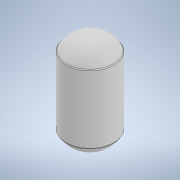
# Autodesk Inventor part: 80. Плунжер стопорный штоков (размер)
Saved by Autodesk Inventor 2021 (Build 250183000, 183)
## iProperties
Created: 2021-03-15
Part Number: 80. Плунжер стопорный штоков (размер)
Material: Типовые
Document SubType Name: Modeling
Designer: Данил
Density: 1 g/cm^3
Appearance: По умолчанию
Author: Данил
Autodesk Inventor part; units mm, degrees
ref_plane "YZ Plane" through (0, 0, 0) normal (1, 0, 0) x (0, 1, 0)
ref_plane "XZ Plane" through (0, 0, 0) normal (0, 1, 0) x (-1, 0, 0)
ref_plane "XY Plane" through (0, 0, 0) normal (0, 0, 1) x (1, 0, 0)
sketch "Эскиз1" plane through (0, 0, 0) normal (0, 0, 1) x (1, 0, 0)
  line L0 (0, 8) -> (0, -8)
  arc A0 (0, -8) -> (3.8971, -5.75) centre (0, -3.5) ccw
  line L1 (3.8971, -5.75) -> (4, -5.5718)
  line L2 (4, -5.5718) -> (4, 5.5718)
  line L3 (4, 5.5718) -> (3.8971, 5.75)
  arc A1 (3.8971, 5.75) -> (0, 8) centre (0, 3.5) ccw
  point P0 (0, 0)
  point P1 (0, 0)
  dimension "d0" = 16
  dimension "d1" = 4.5
  dimension "d2" = 30
  dimension "d3" = 30
  dimension "d4" = 4.5
  dimension "d5" = 8
  constraints: 8 end point, 4 point on circle, 2 centre point, 2 point on line, 2 tangent, 2 vertical, 1 coincident, 1 midpoint
  measures "d0" distance of L0.start L0.end
  measures "d1" radius of A0
  measures "d2" angle of L1 L2
  measures "d3" angle of L2 L3
  measures "d4" radius of A1
  measures "d5" diameter of L2 L0
revolve "Вращение1" add sketch "Эскиз1" angle 360 about axis through (0, 8, 0) along (0, -1, 0)
